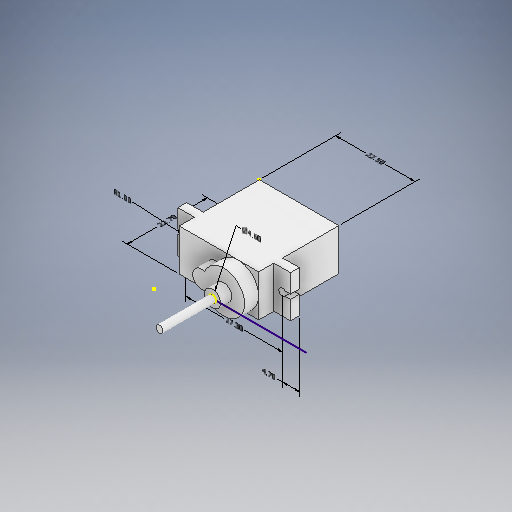
# Autodesk Inventor part: Part1'
Saved by Autodesk Inventor 2025.3 (Build 293356000, 356)
## iProperties
Created: 2026-03-06
Part Number: Part1'
Material: ABS Plastic
Document SubType Name: Modeling
Designer: Youssef Makhlouf
Density: 1.06 g/cm^3
Appearance: Smooth - White
Author: Youssef Makhlouf
Autodesk Inventor part; units mm, degrees
ref_plane "YZ Plane" through (0, 0, 0) normal (1, 0, 0) x (0, 1, 0)
ref_plane "XZ Plane" through (0, 0, 0) normal (0, 1, 0) x (-1, 0, 0)
ref_plane "XY Plane" through (0, 0, 0) normal (0, 0, 1) x (1, 0, 0)
sketch "Sketch1" plane through (0, 0, 0) normal (0, 0, 1) x (1, 0, 0)
  line L0 (0, 0) -> (22.5, 0)
  line L1 (22.5, 0) -> (22.5, 11.8)
  line L2 (22.5, 11.8) -> (0, 11.8)
  line L3 (0, 11.8) -> (0, 0)
  dimension "d6" = 22.5
  dimension "d7" = 11.8
  constraints: 8 end point, 2 parallel, 1 horizontal, 1 perpendicular
  measures "d6" distance of L2.end L1.end
  measures "d7" distance of L1.end L0.end
extrude "Extrusion1" add sketch "Sketch1" along normal blind 22.7
sketch "Sketch2" plane through (0, 0, 22.7) normal (0, 0, 1) x (1, 0, 0)
  circle A0 centre (16.6, 5.9) radius 5.9
  line L0 (22.5, 0) -> (22.5, 11.8) projected
  line L1 (0, 0) -> (22.5, 0) projected
  dimension "d10" = 11.8
  constraints: 2 tangent, 1 centre point
  measures "d10" diameter of A0
extrude "Extrusion2" add sketch "Sketch2" along normal blind 4 contours A0
sketch "Sketch4" plane through (22.5, 0, 0) normal (1, 0, 0) x (0, 0, -1)
  line L0 (0, 11.8) -> (-22.7, 11.8) projected
  line L1 (-18.4, 0) -> (-15.9, 0)
  line L2 (-15.9, 0) -> (-15.9, 11.8)
  line L3 (-15.9, 11.8) -> (-18.4, 11.8)
  line L4 (-18.4, 11.8) -> (-18.4, 0)
  point P0 (0, 0)
  dimension "d16" = 2.5
  dimension "d17" = 15.9
  constraints: 8 end point, 2 parallel, 1 horizontal, 1 perpendicular, 1 point on line
  measures "d16" distance of L3.end L2.end
  measures "d17" distance from line of point (0, 0) L2
extrude "Extrusion4" add sketch "Sketch4" along normal blind 4.7
sketch "Sketch5" plane through (0, 0, 0) normal (-1, 0, 0) x (0, 0, 1)
  line L0 (15.9, 11.8) -> (18.4, 11.8) projected
  line L1 (18.4, 0) -> (15.9, 0) projected
  line L2 (18.4, 11.8) -> (15.9, 11.8)
  line L3 (15.9, 11.8) -> (15.9, 0)
  line L4 (15.9, 0) -> (18.4, 0)
  line L5 (18.4, 0) -> (18.4, 11.8)
  point P0 (0, 0)
  constraints: 8 end point, 2 parallel, 1 horizontal, 1 perpendicular
extrude "Extrusion5" add sketch "Sketch5" along normal blind 4.7
sketch "Sketch6" plane through (22.5, 0, 18.4) normal (0, 0, 1) x (1, 0, 0)
  line L0 (-30.051, 5.9) -> (7.557, 5.9)
  line L1 (-22.5, 0) -> (-27.2, 0) projected
  arc A0 (-25.6599, 5.25) -> (-25.6599, 6.55) centre (-24.9, 5.9) ccw
  line L2 (-27.2, 0) -> (-27.2, 11.8) projected
  line L3 (-27.2, 6.55) -> (-25.6599, 6.55)
  line L4 (-27.2, 5.25) -> (-25.6599, 5.25)
  dimension "d22" = 5.9
  dimension "d23" = 2
  dimension "d24" = 2.3
  dimension "d25" = 1.3
  constraints: 6 end point, 3 horizontal, 3 point on line, 2 point on circle, 1 centre point, 1 other
  measures "d22" distance between parallel lines of L1 L0
  measures "d23" diameter of A0
  measures "d24" distance from line of L2 A0.centre
  measures "d25" distance between parallel lines of L4 L3
extrude "Extrusion6" cut sketch "Sketch6" against normal blind 4.7
sketch "Sketch7" plane through (22.5, 0, 18.4) normal (0, 0, 1) x (1, 0, 0)
  line L0 (0, 0) -> (0, 11.8) projected
  line L1 (0, 0) -> (4.7, 0) projected
  line L2 (4.7, 11.8) -> (4.7, 0) projected
  line L3 (0, 11.8) -> (4.7, 11.8) projected
  arc A0 (3.1599, 6.55) -> (3.1599, 5.25) centre (2.4, 5.9) ccw
  line L4 (3.1599, 6.55) -> (4.7, 6.55)
  line L5 (3.1599, 5.25) -> (4.7, 5.25)
  line L6 (1.0437, 5.9) -> (5.1406, 5.9)
  point P0 (-22.5, 0)
  dimension "d28" = 2
  dimension "d29" = 2.3
  dimension "d30" = 1.3
  dimension "d31" = 11.8
  constraints: 6 end point, 3 point on line, 2 point on circle, 1 centre point, 1 horizontal, 1 parallel, 1 perpendicular, 1 other
  measures "d28" diameter of A0
  measures "d29" distance from line of L2 A0.centre
  measures "d30" distance between parallel lines of L5 L4
  measures "d31" diameter of L1 L6
extrude "Extrusion7" cut sketch "Sketch7" against normal blind 4.7 fills toward (3.93, 5.3) open curves L5 A0 L4
sketch "Sketch8" plane through (16.6, 5.9, 26.7) normal (0, 0, 1) x (1, 0, 0)
  circle A0 centre (-6.3, 0) radius 2.5
  circle A1 centre (0, 0) radius 5.9 projected
  point P0 (-16.6, -5.9)
  point P1 (-5.4167, -2.3387)
  point P2 (-5.4167, 2.3387)
  dimension "d35" = 5
  dimension "d36" = 6.3
  constraints: 1 centre point
  measures "d35" diameter of A0
  measures "d36" distance of A1.centre A0.centre
extrude "Extrusion8" add sketch "Sketch8" against normal blind 4.7 contours A1 A0 picked at (-6.6167, 0.9503)
sketch "Sketch9" plane through (0, 0, 26.7) normal (0, 0, 1) x (1, 0, 0)
  arc A0 (11.1833, 3.5613) -> (11.1833, 8.2387) centre (16.6, 5.9) ccw projected
  arc A1 (11.1833, 8.2387) -> (11.1833, 3.5613) centre (10.3, 5.9) ccw projected
  circle A2 centre (16.6, 5.9) radius 2.3
  point P0 (0, 0)
  dimension "d39" = 4.6
  constraints: 1 centre point, 1 coincident
  measures "d39" diameter of A2
extrude "Extrusion9" add sketch "Sketch9" along normal blind 3.2 contours A2
sketch "Sketch10" plane through (0, 11.8, 0) normal (0, 1, 0) x (1, 0, 0)
  point P0 (0, 0)
sketch "Sketch11" plane through (16.6, 5.9, 29.9) normal (0, 0, 1) x (1, 0, 0)
  circle A0 centre (0, 0) radius 1
  point P0 (-16.6, -5.9)
  dimension "d42" = 2
  constraints: 1 centre point
  measures "d42" diameter of A0
extrude "Extrusion10" add sketch "Sketch11" along normal blind 15
sketch "Sketch12" plane through (16.6, 5.9, 29.9) normal (0, 0, 1) x (1, 0, 0)
  circle A0 centre (0, 0) radius 1 projected
  line L0 (0, 0) -> (26.5658, 0)
  point P0 (-16.6, -5.9)
  constraints: 2 end point, 1 horizontal
body "Solid1"
